Autodesk Inventor part; units mm, degrees
(part 3 of 11)
  arc A664 (23.2868, 30.3149) -> (23.2868, 30.2387) centre (23.2868, 30.2768) ccw
  arc A665 (26.162, 30.2387) -> (26.162, 30.3149) centre (26.162, 30.2768) ccw
  line L333 (27.1241, 30.7326) -> (21.4917, 28.6469)
  arc A666 (21.4537, 28.6494) -> (21.5298, 28.6444) centre (21.4917, 28.6469) ccw
  arc A667 (27.1241, 30.6945) -> (27.1241, 30.7707) centre (27.1241, 30.7326) ccw
  line L334 (26.162, 30.4292) -> (23.5117, 30.4292)
  arc A668 (23.5117, 30.4673) -> (23.5117, 30.3911) centre (23.5117, 30.4292) ccw
  arc A669 (26.162, 30.3911) -> (26.162, 30.4673) centre (26.162, 30.4292) ccw
  line L335 (26.8955, 30.6777) -> (26.7391, 28.3014)
  arc A670 (26.701, 28.3039) -> (26.7771, 28.2989) centre (26.7391, 28.3014) ccw
  arc A671 (26.8955, 30.6396) -> (26.8955, 30.7158) centre (26.8955, 30.6777) ccw
  line L336 (26.162, 30.5816) -> (23.7661, 30.5816)
  arc A672 (23.7661, 30.6197) -> (23.7661, 30.5435) centre (23.7661, 30.5816) ccw
  arc A673 (26.162, 30.5435) -> (26.162, 30.6197) centre (26.162, 30.5816) ccw
  line L337 (26.724, 30.3927) -> (26.587, 28.3115)
  arc A674 (26.549, 28.314) -> (26.625, 28.309) centre (26.587, 28.3115) ccw
  arc A675 (26.724, 30.3546) -> (26.724, 30.4308) centre (26.724, 30.3927) ccw
  line L338 (26.162, 30.734) -> (24.067, 30.734)
  arc A676 (24.067, 30.7721) -> (24.067, 30.6959) centre (24.067, 30.734) ccw
  arc A677 (26.162, 30.6959) -> (26.162, 30.7721) centre (26.162, 30.734) ccw
  line L339 (26.5493, 30.0586) -> (26.4349, 28.3215)
  arc A678 (26.3969, 28.324) -> (26.4729, 28.319) centre (26.4349, 28.3215) ccw
  arc A679 (26.5493, 30.0205) -> (26.5493, 30.0967) centre (26.5493, 30.0586) ccw
  line L340 (26.162, 30.8864) -> (24.4226, 30.8864)
  arc A680 (24.4226, 30.9245) -> (24.4226, 30.8483) centre (24.4226, 30.8864) ccw
  arc A681 (26.162, 30.8483) -> (26.162, 30.9245) centre (26.162, 30.8864) ccw
  line L341 (26.3694, 29.6455) -> (26.2829, 28.3315)
  arc A682 (26.2448, 28.334) -> (26.3209, 28.329) centre (26.2829, 28.3315) ccw
  arc A683 (26.3694, 29.6074) -> (26.3694, 29.6836) centre (26.3694, 29.6455) ccw
  line L342 (26.162, 31.0388) -> (24.8504, 31.0388)
  arc A684 (24.8504, 31.0769) -> (24.8504, 31.0007) centre (24.8504, 31.0388) ccw
  arc A685 (26.162, 31.0007) -> (26.162, 31.0769) centre (26.162, 31.0388) ccw
  line L343 (26.1708, 28.9489) -> (26.1308, 28.3415)
  arc A686 (26.0928, 28.344) -> (26.1688, 28.339) centre (26.1308, 28.3415) ccw
  arc A687 (26.1708, 28.9108) -> (26.1708, 28.987) centre (26.1708, 28.9489) ccw
  line L344 (26.162, 31.1912) -> (25.5924, 31.1912)
  arc A688 (25.5924, 31.2293) -> (25.5924, 31.1531) centre (25.5924, 31.1912) ccw
  arc A689 (26.162, 31.1531) -> (26.162, 31.2293) centre (26.162, 31.1912) ccw
  line L345 (26.0801, 28.3448) -> (26.177, 28.9906)
  arc A690 (26.2147, 28.9849) -> (26.1802, 29.0285) centre (26.177, 28.9906) ccw
  arc A691 (26.0833, 28.3828) -> (26.0769, 28.3069) centre (26.0801, 28.3448) ccw
  line L346 (26.177, 28.9906) -> (26.3574, 29.6181)
  arc A692 (26.394, 29.6076) -> (26.3655, 29.6553) centre (26.3574, 29.6181) ccw
  arc A693 (26.1404, 29.0011) -> (26.1689, 28.9533) centre (26.177, 28.9906) ccw
  line L347 (26.3574, 29.6181) -> (26.6182, 30.2168)
  arc A694 (26.6053, 30.1809) -> (26.6311, 30.2526) centre (26.6182, 30.2168) ccw
  arc A695 (26.3225, 29.6333) -> (26.3445, 29.5823) centre (26.3574, 29.6181) ccw
  line L348 (26.6182, 30.2168) -> (26.9548, 30.7763)
  arc A696 (26.9374, 30.7424) -> (26.9723, 30.8101) centre (26.9548, 30.7763) ccw
  arc A697 (26.6356, 30.2506) -> (26.6007, 30.1829) centre (26.6182, 30.2168) ccw
  line L349 (26.9548, 30.7763) -> (29.3598, 30.1565)
  arc A698 (29.3381, 30.1252) -> (29.3815, 30.1878) centre (29.3598, 30.1565) ccw
  arc A699 (26.9766, 30.8075) -> (26.9331, 30.745) centre (26.9548, 30.7763) ccw
  line L350 (29.3598, 30.1565) -> (29.843, 29.7173)
  arc A700 (29.8174, 29.6891) -> (29.8686, 29.7455) centre (29.843, 29.7173) ccw
  arc A701 (29.3854, 30.1847) -> (29.3342, 30.1283) centre (29.3598, 30.1565) ccw
  line L351 (29.843, 29.7173) -> (30.2647, 29.2188)
  arc A702 (30.2356, 29.1942) -> (30.2938, 29.2434) centre (30.2647, 29.2188) ccw
  arc A703 (29.8721, 29.7419) -> (29.8139, 29.6927) centre (29.843, 29.7173) ccw
  line L352 (30.2647, 29.2188) -> (30.6178, 28.6694)
  arc A704 (30.5857, 28.6489) -> (30.6498, 28.6901) centre (30.6178, 28.6694) ccw
  arc A705 (30.2968, 29.2394) -> (30.2327, 29.1982) centre (30.2647, 29.2188) ccw
  line L353 (30.6178, 28.6694) -> (30.8961, 28.0788)
  arc A706 (30.8616, 28.0625) -> (30.9306, 28.095) centre (30.8961, 28.0788) ccw
  arc A707 (30.6522, 28.6857) -> (30.5833, 28.6532) centre (30.6178, 28.6694) ccw
  line L354 (30.8961, 28.0788) -> (31.0949, 27.4568)
  arc A708 (31.0586, 27.4452) -> (31.1312, 27.4684) centre (31.0949, 27.4568) ccw
  arc A709 (30.9324, 28.0903) -> (30.8598, 28.0672) centre (30.8961, 28.0788) ccw
  line L355 (31.0949, 27.4568) -> (31.2111, 26.8142)
  arc A710 (31.1736, 26.8075) -> (31.2486, 26.821) centre (31.2111, 26.8142) ccw
  arc A711 (31.1324, 27.4636) -> (31.0574, 27.45) centre (31.0949, 27.4568) ccw
  line L356 (31.2111, 26.8142) -> (31.2392, 26.1619)
  arc A712 (31.2012, 26.1601) -> (31.2773, 26.1637) centre (31.2392, 26.1619) ccw
  arc A713 (31.2491, 26.8161) -> (31.173, 26.8124) centre (31.2111, 26.8142) ccw
  line L357 (31.2392, 26.1619) -> (31.2053, 25.5496)
  arc A714 (31.1673, 25.5519) -> (31.2433, 25.5473) centre (31.2053, 25.5496) ccw
  arc A715 (31.2773, 26.1596) -> (31.2012, 26.1642) centre (31.2392, 26.1619) ccw
  line L358 (31.2053, 25.5496) -> (31.0945, 24.9462)
  arc A716 (31.0569, 24.9531) -> (31.1319, 24.9394) centre (31.0944, 24.9463) ccw
  arc A717 (31.2428, 25.5427) -> (31.1678, 25.5565) centre (31.2053, 25.5496) ccw
  line L359 (31.0945, 24.9462) -> (30.9118, 24.3606)
  arc A718 (30.8754, 24.372) -> (30.9482, 24.3493) centre (30.9118, 24.3606) ccw
  arc A719 (31.1309, 24.9349) -> (31.0581, 24.9576) centre (31.0945, 24.9462) ccw
  line L360 (30.9118, 24.3606) -> (30.6601, 23.8012)
  arc A720 (30.6253, 23.8168) -> (30.6948, 23.7856) centre (30.6601, 23.8012) ccw
  arc A721 (30.9465, 24.345) -> (30.877, 24.3763) centre (30.9118, 24.3606) ccw
  line L361 (30.6601, 23.8012) -> (30.3428, 23.2762)
  arc A722 (30.3102, 23.2959) -> (30.3754, 23.2565) centre (30.3428, 23.2762) ccw
  arc A723 (30.6927, 23.7815) -> (30.6275, 23.8209) centre (30.6601, 23.8012) ccw
  line L362 (30.3428, 23.2762) -> (29.9645, 22.7933)
  arc A724 (29.9345, 22.8168) -> (29.9945, 22.7698) centre (29.9645, 22.7933) ccw
  arc A725 (30.3728, 23.2527) -> (30.3128, 23.2997) centre (30.3428, 23.2762) ccw
  line L363 (29.9645, 22.7933) -> (29.5307, 22.3596)
  arc A726 (29.5037, 22.3865) -> (29.5576, 22.3326) centre (29.5307, 22.3596) ccw
  arc A727 (29.9914, 22.7664) -> (29.9375, 22.8203) centre (29.9645, 22.7933) ccw
  line L364 (29.5307, 22.3596) -> (29.0478, 21.9812)
  arc A728 (29.0243, 22.0112) -> (29.0713, 21.9512) centre (29.0478, 21.9812) ccw
  arc A729 (29.5542, 22.3296) -> (29.5072, 22.3896) centre (29.5307, 22.3596) ccw
  line L365 (29.0478, 21.9812) -> (28.5228, 21.6639)
  arc A730 (28.5031, 21.6965) -> (28.5425, 21.6313) centre (28.5228, 21.6639) ccw
  arc A731 (29.0675, 21.9486) -> (29.0281, 22.0138) centre (29.0478, 21.9812) ccw
  line L366 (28.5228, 21.6639) -> (27.9634, 21.4121)
  arc A732 (27.9478, 21.4469) -> (27.9791, 21.3774) centre (27.9634, 21.4121) ccw
  arc A733 (28.5384, 21.6291) -> (28.5072, 21.6986) centre (28.5228, 21.6639) ccw
  line L367 (27.9634, 21.4121) -> (27.3777, 21.2296)
  arc A734 (27.3664, 21.266) -> (27.3891, 21.1933) centre (27.3777, 21.2296) ccw
  arc A735 (27.9747, 21.3758) -> (27.9521, 21.4485) centre (27.9634, 21.4121) ccw
  line L368 (27.3777, 21.2296) -> (26.7743, 21.119)
  arc A736 (26.7675, 21.1565) -> (26.7812, 21.0816) centre (26.7743, 21.119) ccw
  arc A737 (27.3846, 21.1921) -> (27.3709, 21.2671) centre (27.3777, 21.2296) ccw
  line L369 (26.7743, 21.119) -> (26.162, 21.082)
  arc A738 (26.1597, 21.12) -> (26.1643, 21.044) centre (26.162, 21.082) ccw
  arc A739 (26.7766, 21.081) -> (26.772, 21.1571) centre (26.7743, 21.119) ccw
  line L370 (26.162, 21.082) -> (25.5497, 21.119)
  arc A740 (25.552, 21.1571) -> (25.5474, 21.081) centre (25.5497, 21.119) ccw
  arc A741 (26.1597, 21.044) -> (26.1643, 21.12) centre (26.162, 21.082) ccw
  line L371 (25.5497, 21.119) -> (24.9463, 21.2296)
  arc A742 (24.9531, 21.2671) -> (24.9394, 21.1921) centre (24.9463, 21.2296) ccw
  arc A743 (25.5428, 21.0816) -> (25.5565, 21.1565) centre (25.5497, 21.119) ccw
  line L372 (24.9463, 21.2296) -> (24.3606, 21.4121)
  arc A744 (24.3719, 21.4485) -> (24.3493, 21.3758) centre (24.3606, 21.4121) ccw
  arc A745 (24.935, 21.1933) -> (24.9576, 21.266) centre (24.9463, 21.2296) ccw
  line L373 (24.3606, 21.4121) -> (23.8012, 21.6639)
  arc A746 (23.8168, 21.6986) -> (23.7856, 21.6291) centre (23.8012, 21.6639) ccw
  arc A747 (24.345, 21.3774) -> (24.3763, 21.4469) centre (24.3606, 21.4121) ccw
  line L374 (23.8012, 21.6639) -> (23.2762, 21.9812)
  arc A748 (23.2959, 22.0138) -> (23.2565, 21.9486) centre (23.2762, 21.9812) ccw
  arc A749 (23.7815, 21.6313) -> (23.8209, 21.6965) centre (23.8012, 21.6639) ccw
  line L375 (23.2762, 21.9812) -> (22.7933, 22.3596)
  arc A750 (22.8168, 22.3896) -> (22.7698, 22.3296) centre (22.7933, 22.3596) ccw
  arc A751 (23.2527, 21.9512) -> (23.2997, 22.0112) centre (23.2762, 21.9812) ccw
  line L376 (22.7933, 22.3596) -> (22.3596, 22.7933)
  arc A752 (22.3865, 22.8203) -> (22.3326, 22.7664) centre (22.3596, 22.7933) ccw
  arc A753 (22.7664, 22.3326) -> (22.8203, 22.3865) centre (22.7933, 22.3596) ccw
  line L377 (22.3596, 22.7933) -> (21.9812, 23.2762)
  arc A754 (22.0112, 23.2997) -> (21.9512, 23.2527) centre (21.9812, 23.2762) ccw
  arc A755 (22.3296, 22.7698) -> (22.3896, 22.8168) centre (22.3596, 22.7933) ccw
  line L378 (21.9812, 23.2762) -> (21.6639, 23.8012)
  arc A756 (21.6965, 23.8209) -> (21.6313, 23.7815) centre (21.6639, 23.8012) ccw
  arc A757 (21.9486, 23.2565) -> (22.0139, 23.2959) centre (21.9812, 23.2762) ccw
  line L379 (21.6639, 23.8012) -> (21.4121, 24.3606)
  arc A758 (21.4469, 24.3763) -> (21.3774, 24.345) centre (21.4121, 24.3606) ccw
  arc A759 (21.6291, 23.7856) -> (21.6986, 23.8168) centre (21.6639, 23.8012) ccw
  line L380 (21.4121, 24.3606) -> (21.2296, 24.9463)
  arc A760 (21.266, 24.9576) -> (21.1933, 24.935) centre (21.2296, 24.9463) ccw
  arc A761 (21.3758, 24.3493) -> (21.4485, 24.3719) centre (21.4121, 24.3606) ccw
  line L381 (21.2296, 24.9463) -> (21.119, 25.5497)
  arc A762 (21.1565, 25.5565) -> (21.0816, 25.5428) centre (21.119, 25.5497) ccw
  arc A763 (21.1921, 24.9394) -> (21.2671, 24.9531) centre (21.2296, 24.9463) ccw
  line L382 (21.119, 25.5497) -> (21.082, 26.162)
  arc A764 (21.12, 26.1643) -> (21.044, 26.1597) centre (21.082, 26.162) ccw
  arc A765 (21.081, 25.5474) -> (21.1571, 25.552) centre (21.119, 25.5497) ccw
  line L383 (21.082, 26.162) -> (21.1406, 26.8194)
  arc A766 (21.1786, 26.816) -> (21.1027, 26.8228) centre (21.1406, 26.8194) ccw
  arc A767 (21.0441, 26.1654) -> (21.1199, 26.1586) centre (21.082, 26.162) ccw
  line L384 (21.1406, 26.8194) -> (21.2818, 27.464)
  arc A768 (21.319, 27.4559) -> (21.2446, 27.4722) centre (21.2818, 27.464) ccw
  arc A769 (21.1034, 26.8275) -> (21.1778, 26.8112) centre (21.1406, 26.8194) ccw
  line L385 (21.2818, 27.464) -> (21.5033, 28.0857)
  arc A770 (21.5392, 28.073) -> (21.4674, 28.0985) centre (21.5033, 28.0857) ccw
  arc A771 (21.2459, 27.4768) -> (21.3177, 27.4513) centre (21.2818, 27.464) ccw
  line L386 (21.5033, 28.0857) -> (21.8015, 28.6745)
  arc A772 (21.8355, 28.6573) -> (21.7675, 28.6917) centre (21.8015, 28.6745) ccw
  arc A773 (21.4693, 28.103) -> (21.5373, 28.0685) centre (21.5033, 28.0857) ccw
  line L387 (21.8015, 28.6745) -> (22.1716, 29.2209)
  arc A774 (22.2032, 29.1995) -> (22.1401, 29.2422) centre (22.1716, 29.2209) ccw
  arc A775 (21.7699, 28.6959) -> (21.833, 28.6532) centre (21.8015, 28.6745) ccw
  line L388 (22.1716, 29.2209) -> (22.6078, 29.7162)
  arc A776 (22.6364, 29.691) -> (22.5793, 29.7413) centre (22.6078, 29.7162) ccw
  arc A777 (22.143, 29.2461) -> (22.2002, 29.1957) centre (22.1716, 29.2209) ccw
  line L389 (22.6078, 29.7162) -> (23.1031, 30.1524)
  arc A778 (23.1283, 30.1238) -> (23.0779, 30.181) centre (23.1031, 30.1524) ccw
  arc A779 (22.5827, 29.7447) -> (22.633, 29.6876) centre (22.6078, 29.7162) ccw
  line L390 (23.1031, 30.1524) -> (23.6495, 30.5225)
  arc A780 (23.6708, 30.491) -> (23.6281, 30.5541) centre (23.6495, 30.5225) ccw
  arc A781 (23.0817, 30.1839) -> (23.1245, 30.1208) centre (23.1031, 30.1524) ccw
  line L391 (23.6495, 30.5225) -> (24.2383, 30.8207)
  arc A782 (24.2555, 30.7867) -> (24.221, 30.8547) centre (24.2382, 30.8207) ccw
  arc A783 (23.6323, 30.5565) -> (23.6667, 30.4885) centre (23.6495, 30.5225) ccw
  line L392 (24.2383, 30.8207) -> (24.8599, 31.0422)
  arc A784 (24.8727, 31.0063) -> (24.8472, 31.0781) centre (24.8599, 31.0422) ccw
  arc A785 (24.2255, 30.8566) -> (24.251, 30.7848) centre (24.2382, 30.8207) ccw
  line L393 (24.8599, 31.0422) -> (25.5046, 31.1834)
  arc A786 (25.5128, 31.1462) -> (25.4965, 31.2206) centre (25.5046, 31.1834) ccw
  arc A787 (24.8518, 31.0794) -> (24.8681, 31.005) centre (24.8599, 31.0422) ccw
  line L394 (25.5046, 31.1834) -> (26.162, 31.242)
  arc A788 (26.1654, 31.2041) -> (26.1586, 31.28) centre (26.162, 31.242) ccw
  arc A789 (25.5012, 31.2213) -> (25.508, 31.1454) centre (25.5046, 31.1834) ccw
  line L395 (26.162, 31.242) -> (26.162, 29.972)
  arc A790 (26.1239, 29.972) -> (26.2001, 29.972) centre (26.162, 29.972) ccw
  arc A791 (26.2001, 31.242) -> (26.1239, 31.242) centre (26.162, 31.242) ccw
  line L396 (26.162, 29.972) -> (25.6365, 29.9526)
  arc A792 (25.6352, 29.9907) -> (25.638, 29.9145) centre (25.6366, 29.9526) ccw
  arc A793 (26.1634, 29.9339) -> (26.1606, 30.0101) centre (26.162, 29.972) ccw
  line L397 (25.6365, 29.9526) -> (25.1192, 29.8586)
  arc A794 (25.1124, 29.8961) -> (25.126, 29.8211) centre (25.1192, 29.8586) ccw
  arc A795 (25.6434, 29.9151) -> (25.6297, 29.9901) centre (25.6366, 29.9526) ccw
  line L398 (25.1192, 29.8586) -> (24.6206, 29.6919)
  arc A796 (24.6085, 29.7281) -> (24.6326, 29.6558) centre (24.6206, 29.6919) ccw
  arc A797 (25.1313, 29.8225) -> (25.1072, 29.8947) centre (25.1192, 29.8586) ccw
  line L399 (24.6206, 29.6919) -> (24.1507, 29.456)
  arc A798 (24.1336, 29.49) -> (24.1677, 29.4219) centre (24.1506, 29.456) ccw
  arc A799 (24.6376, 29.6579) -> (24.6035, 29.726) centre (24.6206, 29.6919) ccw
  line L400 (24.1507, 29.456) -> (23.7191, 29.1556)
  arc A800 (23.6974, 29.1868) -> (23.7409, 29.1243) centre (23.7191, 29.1556) ccw
  arc A801 (24.1724, 29.4247) -> (24.1289, 29.4873) centre (24.1507, 29.456) ccw
  line L401 (23.7191, 29.1556) -> (23.3348, 28.7968)
  arc A802 (23.3087, 28.8247) -> (23.3607, 28.769) centre (23.3347, 28.7968) ccw
  arc A803 (23.7451, 29.1277) -> (23.6931, 29.1834) centre (23.7191, 29.1556) ccw
  line L402 (23.3348, 28.7968) -> (23.0053, 28.387)
  arc A804 (22.9756, 28.4109) -> (23.035, 28.3631) centre (23.0053, 28.387) ccw
  arc A805 (23.3644, 28.773) -> (23.305, 28.8207) centre (23.3347, 28.7968) ccw
  line L403 (23.0053, 28.387) -> (22.7376, 27.9345)
  arc A806 (22.7048, 27.9539) -> (22.7704, 27.9151) centre (22.7376, 27.9345) ccw
  arc A807 (23.0381, 28.3676) -> (22.9725, 28.4064) centre (23.0053, 28.387) ccw
  line L404 (22.7376, 27.9345) -> (22.5369, 27.4485)
  arc A808 (22.5018, 27.463) -> (22.5722, 27.4339) centre (22.537, 27.4485) ccw
  arc A809 (22.7728, 27.92) -> (22.7024, 27.949) centre (22.7376, 27.9345) ccw
  line L405 (22.5369, 27.4485) -> (22.4076, 26.9389)
  arc A810 (22.3706, 26.9482) -> (22.4445, 26.9295) centre (22.4076, 26.9388) ccw
  arc A811 (22.5739, 27.4391) -> (22.5, 27.4579) centre (22.5369, 27.4485) ccw
  line L406 (22.4076, 26.9389) -> (22.352, 26.416)
  arc A812 (22.3141, 26.42) -> (22.3899, 26.412) centre (22.352, 26.416) ccw
  arc A813 (22.4454, 26.9348) -> (22.3697, 26.9429) centre (22.4076, 26.9388) ccw
  line L407 (22.352, 26.416) -> (22.352, 26.162)
  arc A814 (22.3139, 26.162) -> (22.3901, 26.162) centre (22.352, 26.162) ccw
  arc A815 (22.3901, 26.416) -> (22.3139, 26.416) centre (22.352, 26.416) ccw
  line L408 (22.352, 26.162) -> (22.3908, 25.6198)
  arc A816 (22.3528, 25.6171) -> (22.4288, 25.6225) centre (22.3908, 25.6198) ccw
  arc A817 (22.39, 26.1647) -> (22.314, 26.1593) centre (22.352, 26.162) ccw
  line L409 (22.3908, 25.6198) -> (22.5063, 25.0886)
  arc A818 (22.4691, 25.0805) -> (22.5436, 25.0967) centre (22.5063, 25.0886) ccw
  arc A819 (22.428, 25.6279) -> (22.3536, 25.6117) centre (22.3908, 25.6198) ccw
  line L410 (22.5063, 25.0886) -> (22.6963, 24.5793)
  arc A820 (22.6606, 24.566) -> (22.732, 24.5926) centre (22.6963, 24.5793) ccw
  arc A821 (22.542, 25.1019) -> (22.4706, 25.0753) centre (22.5063, 25.0886) ccw
  line L411 (22.6963, 24.5793) -> (22.9568, 24.1022)
  arc A822 (22.9234, 24.0839) -> (22.9903, 24.1204) centre (22.9568, 24.1022) ccw
  arc A823 (22.7297, 24.5975) -> (22.6629, 24.561) centre (22.6963, 24.5793) ccw
  line L412 (22.9568, 24.1022) -> (23.2827, 23.6671)
  arc A824 (23.2521, 23.6441) -> (23.3131, 23.6898) centre (23.2826, 23.667) ccw
  arc A825 (22.9873, 24.125) -> (22.9263, 24.0793) centre (22.9568, 24.1022) ccw
  line L413 (23.2827, 23.6671) -> (23.667, 23.2826)
  arc A826 (23.64, 23.2557) -> (23.6939, 23.3095) centre (23.667, 23.2826) ccw
  arc A827 (23.3095, 23.6939) -> (23.2557, 23.64) centre (23.2826, 23.667) ccw
  line L414 (23.667, 23.2826) -> (24.1022, 22.9568)
  arc A828 (24.0793, 22.9263) -> (24.125, 22.9873) centre (24.1022, 22.9568) ccw
  arc A829 (23.6898, 23.3131) -> (23.6441, 23.2521) centre (23.667, 23.2826) ccw
  line L415 (24.1022, 22.9568) -> (24.5793, 22.6963)
  arc A830 (24.561, 22.6629) -> (24.5975, 22.7297) centre (24.5793, 22.6963) ccw
  arc A831 (24.1204, 22.9903) -> (24.0839, 22.9234) centre (24.1022, 22.9568) ccw
  line L416 (24.5793, 22.6963) -> (25.0886, 22.5063)
  arc A832 (25.0753, 22.4706) -> (25.1019, 22.542) centre (25.0886, 22.5063) ccw
  arc A833 (24.5926, 22.732) -> (24.566, 22.6606) centre (24.5793, 22.6963) ccw
  line L417 (25.0886, 22.5063) -> (25.6198, 22.3908)
  arc A834 (25.6117, 22.3536) -> (25.6279, 22.428) centre (25.6198, 22.3908) ccw
  arc A835 (25.0967, 22.5436) -> (25.0805, 22.4691) centre (25.0886, 22.5063) ccw
  line L418 (25.6198, 22.3908) -> (26.162, 22.352)
  arc A836 (26.1593, 22.314) -> (26.1647, 22.39) centre (26.162, 22.352) ccw
  arc A837 (25.6225, 22.4288) -> (25.6171, 22.3528) centre (25.6198, 22.3908) ccw
  line L419 (26.162, 22.352) -> (26.7042, 22.3908)
  arc A838 (26.7069, 22.3528) -> (26.7015, 22.4288) centre (26.7042, 22.3908) ccw
  arc A839 (26.1593, 22.39) -> (26.1647, 22.314) centre (26.162, 22.352) ccw
  line L420 (26.7042, 22.3908) -> (27.2354, 22.5063)
  arc A840 (27.2435, 22.4691) -> (27.2273, 22.5436) centre (27.2354, 22.5063) ccw
  arc A841 (26.6961, 22.428) -> (26.7123, 22.3535) centre (26.7042, 22.3908) ccw
  line L421 (27.2354, 22.5063) -> (27.7447, 22.6963)
  arc A842 (27.758, 22.6606) -> (27.7314, 22.732) centre (27.7447, 22.6963) ccw
  arc A843 (27.2221, 22.542) -> (27.2487, 22.4706) centre (27.2354, 22.5063) ccw
  line L422 (27.7447, 22.6963) -> (28.2218, 22.9568)
  arc A844 (28.2401, 22.9234) -> (28.2036, 22.9903) centre (28.2218, 22.9568) ccw
  arc A845 (27.7265, 22.7297) -> (27.763, 22.6629) centre (27.7447, 22.6963) ccw
  line L423 (28.2218, 22.9568) -> (28.657, 23.2826)
  arc A846 (28.6799, 23.2521) -> (28.6342, 23.3131) centre (28.657, 23.2826) ccw
  arc A847 (28.199, 22.9873) -> (28.2447, 22.9263) centre (28.2218, 22.9568) ccw
  line L424 (28.657, 23.2826) -> (29.0414, 23.667)
  arc A848 (29.0683, 23.64) -> (29.0145, 23.6939) centre (29.0414, 23.667) ccw
  arc A849 (28.6301, 23.3095) -> (28.684, 23.2557) centre (28.657, 23.2826) ccw
  line L425 (29.0414, 23.667) -> (29.3672, 24.1022)
  arc A850 (29.3977, 24.0793) -> (29.3367, 24.125) centre (29.3672, 24.1022) ccw
  arc A851 (29.0109, 23.6898) -> (29.0719, 23.6441) centre (29.0414, 23.667) ccw
  line L426 (29.3672, 24.1022) -> (29.6277, 24.5793)
  arc A852 (29.6611, 24.561) -> (29.5943, 24.5975) centre (29.6277, 24.5793) ccw
  arc A853 (29.3337, 24.1204) -> (29.4006, 24.0839) centre (29.3672, 24.1022) ccw
  line L427 (29.6277, 24.5793) -> (29.8177, 25.0886)
  arc A854 (29.8534, 25.0753) -> (29.782, 25.1019) centre (29.8177, 25.0886) ccw
  arc A855 (29.592, 24.5926) -> (29.6634, 24.566) centre (29.6277, 24.5793) ccw
  line L428 (29.8177, 25.0886) -> (29.9332, 25.6198)
  arc A856 (29.9704, 25.6117) -> (29.896, 25.6279) centre (29.9332, 25.6198) ccw
  arc A857 (29.7804, 25.0967) -> (29.8549, 25.0805) centre (29.8177, 25.0886) ccw
  line L429 (29.9332, 25.6198) -> (29.972, 26.162)
  arc A858 (30.01, 26.1593) -> (29.934, 26.1647) centre (29.972, 26.162) ccw
  arc A859 (29.8952, 25.6225) -> (29.9712, 25.6171) centre (29.9332, 25.6198) ccw
  line L430 (29.972, 26.162) -> (29.9518, 26.6485)
  arc A860 (29.9898, 26.65) -> (29.9137, 26.6469) centre (29.9518, 26.6485) ccw
  arc A861 (29.9339, 26.1604) -> (30.0101, 26.1636) centre (29.972, 26.162) ccw
  line L431 (29.9518, 26.6485) -> (29.8682, 27.1281)
  arc A862 (29.9058, 27.1347) -> (29.8307, 27.1216) centre (29.8682, 27.1281) ccw
  arc A863 (29.9142, 26.6419) -> (29.9893, 26.655) centre (29.9518, 26.6485) ccw
  line L432 (29.8682, 27.1281) -> (29.7228, 27.5928)
  arc A864 (29.7591, 27.6042) -> (29.6864, 27.5814) centre (29.7228, 27.5928) ccw
  arc A865 (29.8318, 27.1167) -> (29.9046, 27.1395) centre (29.8682, 27.1281) ccw
  line L433 (29.7228, 27.5928) -> (29.5179, 28.0345)
  arc A866 (29.5525, 28.0505) -> (29.4834, 28.0184) centre (29.5179, 28.0345) ccw
  arc A867 (29.6882, 27.5767) -> (29.7574, 27.6088) centre (29.7228, 27.5928) ccw
  line L434 (29.5179, 28.0345) -> (29.2572, 28.4456)
  arc A868 (29.2893, 28.466) -> (29.225, 28.4252) centre (29.2572, 28.4456) ccw
  arc A869 (29.4857, 28.0141) -> (29.5501, 28.0549) centre (29.5179, 28.0345) ccw
  line L435 (29.2572, 28.4456) -> (28.945, 28.8193)
  arc A870 (28.9742, 28.8437) -> (28.9157, 28.7948) centre (28.945, 28.8193) ccw
  arc A871 (29.2279, 28.4212) -> (29.2864, 28.4701) centre (29.2572, 28.4456) ccw
  line L436 (28.945, 28.8193) -> (28.5867, 29.1489)
  arc A872 (28.6125, 29.177) -> (28.5609, 29.1209) centre (28.5867, 29.1489) ccw
  arc A873 (28.9192, 28.7912) -> (28.9708, 28.8473) centre (28.945, 28.8193) ccw
  line L437 (28.5867, 29.1489) -> (28.1884, 29.429)
  arc A874 (28.2104, 29.4602) -> (28.1665, 29.3979) centre (28.1884, 29.429) ccw
  arc A875 (28.5648, 29.1178) -> (28.6086, 29.1801) centre (28.5867, 29.1489) ccw
  line L438 (28.1884, 29.429) -> (27.757, 29.6547)
  arc A876 (27.7747, 29.6885) -> (27.7394, 29.621) centre (27.757, 29.6547) ccw
  arc A877 (28.1708, 29.3953) -> (28.2061, 29.4628) centre (28.1884, 29.429) ccw
  line L439 (27.757, 29.6547) -> (27.5599, 29.2096)
  arc A878 (27.313, 29.858) -> (27.2868, 29.7864) centre (27.2999, 29.8222) ccw
  arc A879 (27.7439, 29.619) -> (27.7702, 29.6905) centre (27.757, 29.6547) ccw
  line L440 (27.5599, 29.2096) -> (27.4225, 28.7424)
  arc A880 (27.4309, 28.7796) -> (27.4142, 28.7052) centre (27.4225, 28.7424) ccw
  arc A881 (27.5516, 29.1724) -> (27.5682, 29.2467) centre (27.5599, 29.2095) ccw
  line L441 (27.4225, 28.7424) -> (27.3473, 28.2614)
  arc A882 (27.3507, 28.2993) -> (27.3439, 28.2235) centre (27.3473, 28.2614) ccw
  arc A883 (27.4191, 28.7045) -> (27.4259, 28.7804) centre (27.4225, 28.7424) ccw
  line L442 (27.3473, 28.2614) -> (26.0801, 28.3448)
  arc A884 (26.1182, 28.3448) -> (26.042, 28.3448) centre (26.0801, 28.3448) ccw
  arc A885 (27.3092, 28.2614) -> (27.3775, 28.2847) centre (27.3473, 28.2614) ccw
  line L443 (26.8494, 21.1328) -> (25.4746, 21.1328)
  arc A886 (25.4746, 21.1709) -> (25.4746, 21.0947) centre (25.4746, 21.1328) ccw
  arc A887 (26.8494, 21.0947) -> (26.8494, 21.1709) centre (26.8494, 21.1328) ccw
  line L444 (27.5561, 21.2852) -> (24.7679, 21.2852)
  arc A888 (24.7679, 21.3233) -> (24.7679, 21.2471) centre (24.7679, 21.2852) ccw
  arc A889 (27.5561, 21.2471) -> (27.5561, 21.3233) centre (27.5561, 21.2852) ccw
  line L445 (28.02, 21.4376) -> (24.304, 21.4376)
  arc A890 (24.304, 21.4757) -> (24.304, 21.3995) centre (24.304, 21.4376) ccw
  arc A891 (28.02, 21.3995) -> (28.02, 21.4757) centre (28.02, 21.4376) ccw
  line L446 (28.3587, 21.59) -> (23.9654, 21.59)
  arc A892 (23.9654, 21.6281) -> (23.9654, 21.5519) centre (23.9654, 21.59) ccw
  arc A893 (28.3587, 21.5519) -> (28.3587, 21.6281) centre (28.3587, 21.59) ccw
  line L447 (28.6527, 21.7424) -> (23.6713, 21.7424)
  arc A894 (23.6713, 21.7805) -> (23.6713, 21.7043) centre (23.6713, 21.7424) ccw
  arc A895 (28.6527, 21.7043) -> (28.6527, 21.7805) centre (28.6527, 21.7424) ccw
  line L448 (28.9048, 21.8948) -> (23.4192, 21.8948)
  arc A896 (23.4192, 21.9329) -> (23.4192, 21.8567) centre (23.4192, 21.8948) ccw
  arc A897 (28.9048, 21.8567) -> (28.9048, 21.9329) centre (28.9048, 21.8948) ccw
  line L449 (29.132, 22.0472) -> (23.1921, 22.0471)
  arc A898 (23.1921, 22.0852) -> (23.1921, 22.009) centre (23.1921, 22.0471) ccw
  arc A899 (29.132, 22.0091) -> (29.132, 22.0853) centre (29.132, 22.0472) ccw
  line L450 (29.3265, 22.1996) -> (22.9975, 22.1996)
  arc A900 (22.9975, 22.2377) -> (22.9975, 22.1615) centre (22.9975, 22.1996) ccw
  arc A901 (29.3265, 22.1615) -> (29.3265, 22.2377) centre (29.3265, 22.1996) ccw
  line L451 (29.521, 22.352) -> (26.162, 22.352)
  arc A902 (26.162, 22.3901) -> (26.162, 22.3139) centre (26.162, 22.352) ccw
  arc A903 (29.521, 22.3139) -> (29.521, 22.3901) centre (29.521, 22.352) ccw
  line L452 (26.162, 22.352) -> (22.803, 22.352)
  arc A904 (22.803, 22.3901) -> (22.803, 22.3139) centre (22.803, 22.352) ccw
  arc A905 (26.162, 22.3139) -> (26.162, 22.3901) centre (26.162, 22.352) ccw
  line L453 (29.6755, 22.5044) -> (27.2265, 22.5044)
  arc A906 (27.2265, 22.5425) -> (27.2265, 22.4663) centre (27.2265, 22.5044) ccw
  arc A907 (29.6755, 22.4663) -> (29.6755, 22.5425) centre (29.6755, 22.5044) ccw
  line L454 (25.0975, 22.5044) -> (22.6485, 22.5044)
  arc A908 (22.6485, 22.5425) -> (22.6485, 22.4663) centre (22.6485, 22.5044) ccw
  arc A909 (25.0975, 22.4663) -> (25.0975, 22.5425) centre (25.0975, 22.5044) ccw
  line L455 (29.8279, 22.6568) -> (27.6388, 22.6568)
  arc A910 (27.6388, 22.6949) -> (27.6388, 22.6187) centre (27.6388, 22.6568) ccw
  arc A911 (29.8279, 22.6187) -> (29.8279, 22.6949) centre (29.8279, 22.6568) ccw
  line L456 (24.6852, 22.6568) -> (22.4961, 22.6568)
  arc A912 (22.4961, 22.6949) -> (22.4961, 22.6187) centre (22.4961, 22.6568) ccw
  arc A913 (24.6852, 22.6187) -> (24.6852, 22.6949) centre (24.6852, 22.6568) ccw
  line L457 (29.9769, 22.8092) -> (27.9515, 22.8092)
  arc A914 (27.9515, 22.8473) -> (27.9515, 22.7711) centre (27.9515, 22.8092) ccw
  arc A915 (29.9769, 22.7711) -> (29.9769, 22.8473) centre (29.9769, 22.8092) ccw
  line L458 (24.3725, 22.8092) -> (22.3471, 22.8092)
  arc A916 (22.3471, 22.8473) -> (22.3471, 22.7711) centre (22.3471, 22.8092) ccw
  arc A917 (24.3725, 22.7711) -> (24.3725, 22.8473) centre (24.3725, 22.8092) ccw
  line L459 (30.0963, 22.9616) -> (28.2282, 22.9616)
  arc A918 (28.2282, 22.9997) -> (28.2282, 22.9235) centre (28.2282, 22.9616) ccw
  arc A919 (30.0963, 22.9235) -> (30.0963, 22.9997) centre (30.0963, 22.9616) ccw
  line L460 (24.0958, 22.9616) -> (22.2277, 22.9616)
  arc A920 (22.2277, 22.9997) -> (22.2277, 22.9235) centre (22.2277, 22.9616) ccw
  arc A921 (24.0958, 22.9235) -> (24.0958, 22.9997) centre (24.0958, 22.9616) ccw
  line L461 (30.2157, 23.114) -> (28.4318, 23.114)
  arc A922 (28.4318, 23.1521) -> (28.4318, 23.0759) centre (28.4318, 23.114) ccw
  arc A923 (30.2157, 23.0759) -> (30.2157, 23.1521) centre (30.2157, 23.114) ccw
  line L462 (23.8922, 23.114) -> (22.1083, 23.114)
  arc A924 (22.1083, 23.1521) -> (22.1083, 23.0759) centre (22.1083, 23.114) ccw
  arc A925 (23.8922, 23.0759) -> (23.8922, 23.1521) centre (23.8922, 23.114) ccw
  line L463 (30.3351, 23.2664) -> (28.6354, 23.2664)
  arc A926 (28.6354, 23.3045) -> (28.6354, 23.2283) centre (28.6354, 23.2664) ccw
  arc A927 (30.3351, 23.2283) -> (30.3351, 23.3045) centre (30.3351, 23.2664) ccw
  line L464 (23.6886, 23.2664) -> (21.9889, 23.2664)
  arc A928 (21.9889, 23.3045) -> (21.9889, 23.2283) centre (21.9889, 23.2664) ccw
  arc A929 (23.6886, 23.2283) -> (23.6886, 23.3045) centre (23.6886, 23.2664) ccw
  line L465 (30.429, 23.4188) -> (28.7933, 23.4186)
  arc A930 (28.7933, 23.4567) -> (28.7933, 23.3805) centre (28.7933, 23.4186) ccw
  arc A931 (30.429, 23.3807) -> (30.429, 23.4569) centre (30.429, 23.4188) ccw
  line L466 (23.5308, 23.4188) -> (21.8951, 23.4188)
  arc A932 (21.8951, 23.4569) -> (21.8951, 23.3807) centre (21.8951, 23.4188) ccw
  arc A933 (23.5308, 23.3807) -> (23.5308, 23.4569) centre (23.5308, 23.4188) ccw
  line L467 (30.5211, 23.5712) -> (28.9456, 23.571)
  arc A934 (28.9456, 23.6091) -> (28.9456, 23.5329) centre (28.9456, 23.571) ccw
  arc A935 (30.5211, 23.5331) -> (30.5211, 23.6093) centre (30.5211, 23.5712) ccw
  line L468 (23.3784, 23.5712) -> (21.8029, 23.5712)
  arc A936 (21.8029, 23.6093) -> (21.8029, 23.5331) centre (21.8029, 23.5712) ccw
  arc A937 (23.3784, 23.5331) -> (23.3784, 23.6093) centre (23.3784, 23.5712) ccw
  line L469 (30.6132, 23.7236) -> (29.0838, 23.7236)
  arc A938 (29.0838, 23.7617) -> (29.0838, 23.6855) centre (29.0838, 23.7236) ccw
  arc A939 (30.6132, 23.6855) -> (30.6132, 23.7617) centre (30.6132, 23.7236) ccw
  line L470 (23.2403, 23.7237) -> (21.7108, 23.7236)
  arc A940 (21.7108, 23.7617) -> (21.7108, 23.6855) centre (21.7108, 23.7236) ccw
  arc A941 (23.2403, 23.6856) -> (23.2403, 23.7618) centre (23.2403, 23.7237) ccw
  line L471 (30.6937, 23.876) -> (29.1979, 23.8758)
  arc A942 (29.1979, 23.9139) -> (29.1979, 23.8377) centre (29.1979, 23.8758) ccw
  arc A943 (30.6937, 23.8379) -> (30.6937, 23.9141) centre (30.6937, 23.876) ccw
  line L472 (23.1261, 23.876) -> (21.6302, 23.876)
  arc A944 (21.6302, 23.9141) -> (21.6302, 23.8379) centre (21.6302, 23.876) ccw
  arc A945 (23.1261, 23.8379) -> (23.1261, 23.9141) centre (23.1261, 23.876) ccw
  line L473 (30.7623, 24.0284) -> (29.312, 24.0284)
  arc A946 (29.312, 24.0665) -> (29.312, 23.9903) centre (29.312, 24.0284) ccw
  arc A947 (30.7623, 23.9903) -> (30.7623, 24.0665) centre (30.7623, 24.0284) ccw
  arc A948 (21.5616, 24.0665) -> (21.5616, 23.9903) centre (21.5616, 24.0284) ccw
  arc A949 (23.0121, 23.9903) -> (23.0121, 24.0665) centre (23.0121, 24.0284) ccw
  line L474 (30.8309, 24.1808) -> (29.4101, 24.1808)
  arc A950 (29.4101, 24.2189) -> (29.4101, 24.1427) centre (29.4101, 24.1808) ccw
  arc A951 (30.8309, 24.1427) -> (30.8309, 24.2189) centre (30.8309, 24.1808) ccw
  line L475 (22.9139, 24.1808) -> (21.4931, 24.1808)
  arc A952 (21.4931, 24.2189) -> (21.4931, 24.1427) centre (21.4931, 24.1808) ccw
  arc A953 (22.9139, 24.1427) -> (22.9139, 24.2189) centre (22.9139, 24.1808) ccw
  line L476 (30.8996, 24.3332) -> (29.4933, 24.3332)
  arc A954 (29.4933, 24.3713) -> (29.4933, 24.2951) centre (29.4933, 24.3332) ccw
  arc A955 (30.8996, 24.2951) -> (30.8996, 24.3713) centre (30.8996, 24.3332) ccw
  line L477 (22.8307, 24.3332) -> (21.4245, 24.3332)
  arc A956 (21.4245, 24.3713) -> (21.4245, 24.2951) centre (21.4245, 24.3332) ccw
  arc A957 (22.8307, 24.2951) -> (22.8307, 24.3713) centre (22.8307, 24.3332) ccw
  line L478 (30.9508, 24.4856) -> (29.5765, 24.4856)
  arc A958 (29.5765, 24.5237) -> (29.5765, 24.4475) centre (29.5765, 24.4856) ccw
  arc A959 (30.9508, 24.4475) -> (30.9508, 24.5237) centre (30.9508, 24.4856) ccw
  line L479 (22.7474, 24.4856) -> (21.3732, 24.4857)
  arc A960 (21.3732, 24.5238) -> (21.3732, 24.4476) centre (21.3732, 24.4857) ccw
  arc A961 (22.7474, 24.4475) -> (22.7474, 24.5237) centre (22.7474, 24.4856) ccw
  line L480 (30.9983, 24.638) -> (29.6496, 24.638)
  arc A962 (29.6496, 24.6761) -> (29.6496, 24.5999) centre (29.6496, 24.638) ccw
  arc A963 (30.9983, 24.5999) -> (30.9983, 24.6761) centre (30.9983, 24.638) ccw
  line L481 (22.6744, 24.638) -> (21.3257, 24.638)
  arc A964 (21.3257, 24.6761) -> (21.3257, 24.5999) centre (21.3257, 24.638) ccw
  arc A965 (22.6744, 24.5999) -> (22.6744, 24.6761) centre (22.6744, 24.638) ccw
  line L482 (31.0459, 24.7904) -> (29.7064, 24.7904)
  arc A966 (29.7064, 24.8285) -> (29.7064, 24.7523) centre (29.7064, 24.7904) ccw
  arc A967 (31.0459, 24.7523) -> (31.0459, 24.8285) centre (31.0459, 24.7904) ccw
  line L483 (22.6176, 24.7904) -> (21.2782, 24.7904)
  arc A968 (21.2782, 24.8285) -> (21.2782, 24.7523) centre (21.2782, 24.7904) ccw
  arc A969 (22.6176, 24.7523) -> (22.6176, 24.8285) centre (22.6176, 24.7904) ccw
  line L484 (31.0933, 24.9428) -> (29.7633, 24.9428)
  arc A970 (29.7633, 24.9809) -> (29.7633, 24.9047) centre (29.7633, 24.9428) ccw
  arc A971 (31.0933, 24.9047) -> (31.0933, 24.9809) centre (31.0933, 24.9428) ccw
  line L485 (22.5607, 24.9428) -> (21.2307, 24.9428)
  arc A972 (21.2307, 24.9809) -> (21.2307, 24.9047) centre (21.2307, 24.9428) ccw
  arc A973 (22.5607, 24.9047) -> (22.5607, 24.9809) centre (22.5607, 24.9428) ccw
  line L486 (31.1217, 25.0952) -> (29.8191, 25.0952)
  arc A974 (29.8191, 25.1333) -> (29.8191, 25.0571) centre (29.8191, 25.0952) ccw
  arc A975 (31.1217, 25.0571) -> (31.1217, 25.1333) centre (31.1217, 25.0952) ccw
  line L487 (22.5049, 25.0952) -> (21.2023, 25.0952)
  arc A976 (21.2023, 25.1333) -> (21.2023, 25.0571) centre (21.2023, 25.0952) ccw
  arc A977 (22.5049, 25.0571) -> (22.5049, 25.1333) centre (22.5049, 25.0952) ccw
  line L488 (31.1498, 25.2475) -> (29.8523, 25.2476)
  arc A978 (29.8523, 25.2857) -> (29.8523, 25.2095) centre (29.8523, 25.2476) ccw
  arc A979 (31.1498, 25.2094) -> (31.1498, 25.2856) centre (31.1498, 25.2475) ccw
  line L489 (22.4717, 25.2476) -> (21.1744, 25.2476)
  arc A980 (21.1744, 25.2857) -> (21.1744, 25.2095) centre (21.1744, 25.2476) ccw
  arc A981 (22.4717, 25.2095) -> (22.4717, 25.2857) centre (22.4717, 25.2476) ccw
  line L490 (31.1778, 25.3999) -> (29.8854, 25.4)
  arc A982 (29.8854, 25.4381) -> (29.8854, 25.3619) centre (29.8854, 25.4) ccw
  arc A983 (31.1778, 25.3618) -> (31.1778, 25.438) centre (31.1778, 25.3999) ccw
  line L491 (22.4386, 25.4) -> (21.1465, 25.4)
  arc A984 (21.1465, 25.4381) -> (21.1465, 25.3619) centre (21.1465, 25.4) ccw
  arc A985 (22.4386, 25.3619) -> (22.4386, 25.4381) centre (22.4386, 25.4) ccw
  line L492 (31.2051, 25.5524) -> (29.9186, 25.5524)
  arc A986 (29.9186, 25.5905) -> (29.9186, 25.5143) centre (29.9186, 25.5524) ccw
  arc A987 (31.2051, 25.5143) -> (31.2051, 25.5905) centre (31.2051, 25.5524) ccw
  line L493 (22.4054, 25.5524) -> (21.1189, 25.5524)
  arc A988 (21.1189, 25.5905) -> (21.1189, 25.5143) centre (21.1189, 25.5524) ccw
  arc A989 (22.4054, 25.5143) -> (22.4054, 25.5905) centre (22.4054, 25.5524) ccw
  line L494 (31.2139, 25.7047) -> (29.9389, 25.6983)
  arc A990 (29.9389, 25.7364) -> (29.9389, 25.6602) centre (29.9389, 25.6983) ccw
  arc A991 (31.2139, 25.6666) -> (31.2139, 25.7428) centre (31.2139, 25.7047) ccw
  line L495 (22.3847, 25.7048) -> (21.1097, 25.7048)
  arc A992 (21.1097, 25.7429) -> (21.1097, 25.6667) centre (21.1097, 25.7048) ccw
  arc A993 (22.3847, 25.6667) -> (22.3847, 25.7429) centre (22.3847, 25.7048) ccw
  line L496 (31.2224, 25.8572) -> (29.9502, 25.8572)
  arc A994 (29.9502, 25.8953) -> (29.9502, 25.8191) centre (29.9502, 25.8572) ccw
  arc A995 (31.2224, 25.8191) -> (31.2224, 25.8953) centre (31.2224, 25.8572) ccw
  line L497 (22.3738, 25.8572) -> (21.1004, 25.8572)
  arc A996 (21.1004, 25.8953) -> (21.1004, 25.8191) centre (21.1004, 25.8572) ccw
  arc A997 (22.3738, 25.8191) -> (22.3738, 25.8953) centre (22.3738, 25.8572) ccw
  line L498 (31.2308, 26.0096) -> (29.9611, 26.0096)
  arc A998 (29.9611, 26.0477) -> (29.9611, 25.9715) centre (29.9611, 26.0096) ccw
  arc A999 (31.2308, 25.9715) -> (31.2308, 26.0477) centre (31.2308, 26.0096) ccw
  line L499 (22.3629, 26.0096) -> (21.0912, 26.0096)
  arc A1000 (21.0912, 26.0477) -> (21.0912, 25.9715) centre (21.0912, 26.0096) ccw
  arc A1001 (22.3629, 25.9715) -> (22.3629, 26.0477) centre (22.3629, 26.0096) ccw
  line L500 (31.2392, 26.1619) -> (29.972, 26.162)
  arc A1002 (29.972, 26.2001) -> (29.972, 26.1239) centre (29.972, 26.162) ccw
  arc A1003 (31.2392, 26.1238) -> (31.2392, 26.2) centre (31.2392, 26.1619) ccw
  line L501 (22.352, 26.162) -> (21.082, 26.162)
  arc A1004 (21.082, 26.2001) -> (21.082, 26.1239) centre (21.082, 26.162) ccw
  arc A1005 (22.352, 26.1239) -> (22.352, 26.2001) centre (22.352, 26.162) ccw
  line L502 (31.2327, 26.3143) -> (29.9657, 26.3144)
  arc A1006 (29.9657, 26.3525) -> (29.9657, 26.2763) centre (29.9657, 26.3144) ccw
  arc A1007 (31.2327, 26.2762) -> (31.2327, 26.3524) centre (31.2327, 26.3143) ccw
  line L503 (22.352, 26.3144) -> (21.0956, 26.3144)
  arc A1008 (21.0956, 26.3525) -> (21.0956, 26.2763) centre (21.0956, 26.3144) ccw
  arc A1009 (22.352, 26.2763) -> (22.352, 26.3525) centre (22.352, 26.3144) ccw
  line L504 (31.2261, 26.4667) -> (29.9593, 26.4668)
  arc A1010 (29.9593, 26.5049) -> (29.9593, 26.4287) centre (29.9593, 26.4668) ccw
  arc A1011 (31.2261, 26.4286) -> (31.2261, 26.5048) centre (31.2261, 26.4667) ccw
  line L505 (22.3574, 26.4668) -> (21.1092, 26.4668)
  arc A1012 (21.1092, 26.5049) -> (21.1092, 26.4287) centre (21.1092, 26.4668) ccw
  arc A1013 (22.3574, 26.4287) -> (22.3574, 26.5049) centre (22.3574, 26.4668) ccw
  line L506 (31.2195, 26.6192) -> (29.953, 26.6192)
  arc A1014 (29.953, 26.6573) -> (29.953, 26.5811) centre (29.953, 26.6192) ccw
  arc A1015 (31.2195, 26.5811) -> (31.2195, 26.6573) centre (31.2195, 26.6192) ccw
  line L507 (22.3736, 26.6192) -> (21.1228, 26.6192)
  arc A1016 (21.1228, 26.6573) -> (21.1228, 26.5811) centre (21.1228, 26.6192) ccw
  arc A1017 (22.3736, 26.5811) -> (22.3736, 26.6573) centre (22.3736, 26.6192) ccw
  line L508 (31.2129, 26.7716) -> (29.9303, 26.7716)
  arc A1018 (29.9303, 26.8097) -> (29.9303, 26.7335) centre (29.9303, 26.7716) ccw
  arc A1019 (31.2129, 26.7335) -> (31.2129, 26.8097) centre (31.2129, 26.7716) ccw
  line L509 (22.3898, 26.7716) -> (21.1364, 26.7716)
  arc A1020 (21.1364, 26.8097) -> (21.1364, 26.7335) centre (21.1364, 26.7716) ccw
  arc A1021 (22.3898, 26.7335) -> (22.3898, 26.8097) centre (22.3898, 26.7716) ccw
  line L510 (31.1912, 26.924) -> (29.9038, 26.924)
  arc A1022 (29.9038, 26.9621) -> (29.9038, 26.8859) centre (29.9038, 26.924) ccw
  arc A1023 (31.1912, 26.8859) -> (31.1912, 26.9621) centre (31.1912, 26.924) ccw
  line L511 (22.406, 26.924) -> (21.1635, 26.924)
  arc A1024 (21.1635, 26.9621) -> (21.1635, 26.8859) centre (21.1635, 26.924) ccw
  arc A1025 (22.406, 26.8859) -> (22.406, 26.9621) centre (22.406, 26.924) ccw
  line L512 (31.1637, 27.0764) -> (29.8772, 27.0764)
  arc A1026 (29.8772, 27.1145) -> (29.8772, 27.0383) centre (29.8772, 27.0764) ccw
  arc A1027 (31.1637, 27.0383) -> (31.1637, 27.1145) centre (31.1637, 27.0764) ccw
  line L513 (22.4425, 27.0764) -> (21.1969, 27.0764)
  arc A1028 (21.1969, 27.1145) -> (21.1969, 27.0383) centre (21.1969, 27.0764) ccw
  arc A1029 (22.4425, 27.0383) -> (22.4425, 27.1145) centre (22.4425, 27.0764) ccw
  line L514 (31.1361, 27.2288) -> (29.8367, 27.2288)
  arc A1030 (29.8367, 27.2669) -> (29.8367, 27.1907) centre (29.8367, 27.2288) ccw
  arc A1031 (31.1361, 27.1907) -> (31.1361, 27.2669) centre (31.1361, 27.2288) ccw
  line L515 (22.4812, 27.2288) -> (21.2303, 27.2288)
  arc A1032 (21.2303, 27.2669) -> (21.2303, 27.1907) centre (21.2303, 27.2288) ccw
  arc A1033 (22.4812, 27.1907) -> (22.4812, 27.2669) centre (22.4812, 27.2288) ccw
  line L516 (31.1086, 27.3812) -> (29.789, 27.3812)
  arc A1034 (29.789, 27.4193) -> (29.789, 27.3431) centre (29.789, 27.3812) ccw
  arc A1035 (31.1086, 27.3431) -> (31.1086, 27.4193) centre (31.1086, 27.3812) ccw
  line L517 (22.5199, 27.3812) -> (21.2637, 27.3812)
  arc A1036 (21.2637, 27.4193) -> (21.2637, 27.3431) centre (21.2637, 27.3812) ccw
  arc A1037 (22.5199, 27.3431) -> (22.5199, 27.4193) centre (22.5199, 27.3812) ccw
  line L518 (31.0704, 27.5336) -> (29.7413, 27.5336)
  arc A1038 (29.7413, 27.5717) -> (29.7413, 27.4955) centre (29.7413, 27.5336) ccw
  arc A1039 (31.0704, 27.4955) -> (31.0704, 27.5717) centre (31.0704, 27.5336) ccw
  line L519 (22.5721, 27.5336) -> (21.3066, 27.5336)
  arc A1040 (21.3066, 27.5717) -> (21.3066, 27.4955) centre (21.3066, 27.5336) ccw
  arc A1041 (22.5721, 27.4955) -> (22.5721, 27.5717) centre (22.5721, 27.5336) ccw
  line L520 (31.0217, 27.686) -> (29.6795, 27.686)
  arc A1042 (29.6795, 27.7241) -> (29.6795, 27.6479) centre (29.6795, 27.686) ccw
  arc A1043 (31.0217, 27.6479) -> (31.0217, 27.7241) centre (31.0217, 27.686) ccw
  line L521 (22.635, 27.686) -> (21.3609, 27.686)
  arc A1044 (21.3609, 27.7241) -> (21.3609, 27.6479) centre (21.3609, 27.686) ccw
  arc A1045 (22.635, 27.6479) -> (22.635, 27.7241) centre (22.635, 27.686) ccw
  line L522 (30.9729, 27.8384) -> (29.6089, 27.8384)
  arc A1046 (29.6089, 27.8765) -> (29.6089, 27.8003) centre (29.6089, 27.8384) ccw
  arc A1047 (30.9729, 27.8003) -> (30.9729, 27.8765) centre (30.9729, 27.8384) ccw
  line L523 (22.6979, 27.8384) -> (21.4152, 27.8384)
  arc A1048 (21.4152, 27.8765) -> (21.4152, 27.8003) centre (21.4152, 27.8384) ccw
  arc A1049 (22.6979, 27.8003) -> (22.6979, 27.8765) centre (22.6979, 27.8384) ccw
  line L524 (30.9242, 27.9908) -> (29.5382, 27.9908)
  arc A1050 (29.5382, 28.0289) -> (29.5382, 27.9527) centre (29.5382, 27.9908) ccw
  arc A1051 (30.9242, 27.9527) -> (30.9242, 28.0289) centre (30.9242, 27.9908) ccw
  line L525 (22.7709, 27.9908) -> (21.4694, 27.9908)
  arc A1052 (21.4694, 28.0289) -> (21.4694, 27.9527) centre (21.4694, 27.9908) ccw
  arc A1053 (22.7709, 27.9527) -> (22.7709, 28.0289) centre (22.7709, 27.9908) ccw
  line L526 (30.8658, 28.1432) -> (29.449, 28.1432)
  arc A1054 (29.449, 28.1813) -> (29.449, 28.1051) centre (29.449, 28.1432) ccw
  arc A1055 (30.8658, 28.1051) -> (30.8658, 28.1813) centre (30.8658, 28.1432) ccw
  line L527 (22.8611, 28.1432) -> (21.5324, 28.1432)
  arc A1056 (21.5324, 28.1813) -> (21.5324, 28.1051) centre (21.5324, 28.1432) ccw
  arc A1057 (22.8611, 28.1051) -> (22.8611, 28.1813) centre (22.8611, 28.1432) ccw
  line L528 (30.7939, 28.2956) -> (29.3523, 28.2956)
  arc A1058 (29.3523, 28.3337) -> (29.3523, 28.2575) centre (29.3523, 28.2956) ccw
  arc A1059 (30.7939, 28.2575) -> (30.7939, 28.3337) centre (30.7939, 28.2956) ccw
  line L529 (22.9512, 28.2956) -> (21.6096, 28.2956)
  arc A1060 (21.6096, 28.3337) -> (21.6096, 28.2575) centre (21.6096, 28.2956) ccw
  arc A1061 (22.9512, 28.2575) -> (22.9512, 28.3337) centre (22.9512, 28.2956) ccw
  line L530 (30.7221, 28.448) -> (29.2552, 28.448)
  arc A1062 (29.2552, 28.4861) -> (29.2552, 28.4099) centre (29.2552, 28.448) ccw
  arc A1063 (30.7221, 28.4099) -> (30.7221, 28.4861) centre (30.7221, 28.448) ccw
  line L531 (23.0543, 28.448) -> (21.6867, 28.448)
  arc A1064 (21.6867, 28.4861) -> (21.6867, 28.4099) centre (21.6867, 28.448) ccw
  arc A1065 (23.0543, 28.4099) -> (23.0543, 28.4861) centre (23.0543, 28.448) ccw
  line L532 (30.6503, 28.6004) -> (29.1278, 28.6004)
  arc A1066 (29.1278, 28.6385) -> (29.1278, 28.5623) centre (29.1278, 28.6004) ccw
  arc A1067 (30.6503, 28.5623) -> (30.6503, 28.6385) centre (30.6503, 28.6004) ccw
  line L533 (23.1768, 28.6004) -> (21.7639, 28.6004)
  arc A1068 (21.7639, 28.6385) -> (21.7639, 28.5623) centre (21.7639, 28.6004) ccw
  arc A1069 (23.1768, 28.5623) -> (23.1768, 28.6385) centre (23.1768, 28.6004) ccw
  line L534 (30.5642, 28.7528) -> (29.0005, 28.7528)
  arc A1070 (29.0005, 28.7909) -> (29.0005, 28.7147) centre (29.0005, 28.7528) ccw
  arc A1071 (30.5642, 28.7147) -> (30.5642, 28.7909) centre (30.5642, 28.7528) ccw
  line L535 (23.2993, 28.7528) -> (21.8545, 28.7528)
  arc A1072 (21.8545, 28.7909) -> (21.8545, 28.7147) centre (21.8545, 28.7528) ccw
  arc A1073 (23.2993, 28.7147) -> (23.2993, 28.7909) centre (23.2993, 28.7528) ccw
  line L536 (30.4663, 28.9052) -> (28.8516, 28.9052)
  arc A1074 (28.8516, 28.9433) -> (28.8516, 28.8671) centre (28.8516, 28.9052) ccw
  arc A1075 (30.4663, 28.8671) -> (30.4663, 28.9433) centre (30.4663, 28.9052) ccw
  line L537 (23.4509, 28.9052) -> (21.9577, 28.9052)
  arc A1076 (21.9577, 28.9433) -> (21.9577, 28.8671) centre (21.9577, 28.9052) ccw
  arc A1077 (23.4509, 28.8671) -> (23.4509, 28.9433) centre (23.4509, 28.9052) ccw
  line L538 (30.3683, 29.0576) -> (28.6859, 29.0576)
  arc A1078 (28.6859, 29.0957) -> (28.6859, 29.0195) centre (28.6859, 29.0576) ccw
  arc A1079 (30.3683, 29.0195) -> (30.3683, 29.0957) centre (30.3683, 29.0576) ccw
  line L539 (23.6141, 29.0576) -> (22.061, 29.0576)
  arc A1080 (22.061, 29.0957) -> (22.061, 29.0195) centre (22.061, 29.0576) ccw
  arc A1081 (23.6141, 29.0195) -> (23.6141, 29.0957) centre (23.6141, 29.0576) ccw
  line L540 (30.2703, 29.21) -> (28.4999, 29.21)
  arc A1082 (28.4999, 29.2481) -> (28.4999, 29.1719) centre (28.4999, 29.21) ccw
  arc A1083 (30.2703, 29.1719) -> (30.2703, 29.2481) centre (30.2703, 29.21) ccw
  line L541 (23.7973, 29.21) -> (22.1643, 29.21)
  arc A1084 (22.1643, 29.2481) -> (22.1643, 29.1719) centre (22.1643, 29.21) ccw
  arc A1085 (23.7973, 29.1719) -> (23.7973, 29.2481) centre (23.7973, 29.21) ccw
  line L542 (30.1432, 29.3624) -> (28.2832, 29.3624)
  arc A1086 (28.2832, 29.4005) -> (28.2832, 29.3243) centre (28.2832, 29.3624) ccw
  arc A1087 (30.1432, 29.3243) -> (30.1432, 29.4005) centre (30.1432, 29.3624) ccw
  line L543 (24.0162, 29.3624) -> (22.2963, 29.3624)
  arc A1088 (22.2963, 29.4005) -> (22.2963, 29.3243) centre (22.2963, 29.3624) ccw
  arc A1089 (24.0162, 29.3243) -> (24.0162, 29.4005) centre (24.0162, 29.3624) ccw
  line L544 (30.0143, 29.5148) -> (28.0245, 29.5148)
  arc A1090 (28.0245, 29.5529) -> (28.0245, 29.4767) centre (28.0245, 29.5148) ccw
  arc A1091 (30.0143, 29.4767) -> (30.0143, 29.5529) centre (30.0143, 29.5148) ccw
  line L545 (24.2678, 29.5148) -> (22.4305, 29.5148)
  arc A1092 (22.4305, 29.5529) -> (22.4305, 29.4767) centre (22.4305, 29.5148) ccw
  arc A1093 (24.2678, 29.4767) -> (24.2678, 29.5529) centre (24.2678, 29.5148) ccw
  line L546 (29.8854, 29.6672) -> (27.7423, 29.6216)
  arc A1094 (27.7423, 29.6597) -> (27.7423, 29.5835) centre (27.7423, 29.6216) ccw
  arc A1095 (29.8854, 29.6291) -> (29.8854, 29.7053) centre (29.8854, 29.6672) ccw
  line L547 (24.5713, 29.6672) -> (22.5647, 29.6672)
  arc A1096 (22.5647, 29.7053) -> (22.5647, 29.6291) centre (22.5647, 29.6672) ccw
  arc A1097 (24.5713, 29.6291) -> (24.5713, 29.7053) centre (24.5713, 29.6672) ccw
  line L548 (29.7304, 29.8196) -> (27.563, 29.2165)
  arc A1098 (27.563, 29.2546) -> (27.563, 29.1784) centre (27.563, 29.2165) ccw
  arc A1099 (29.7304, 29.7815) -> (29.7304, 29.8577) centre (29.7304, 29.8196) ccw
  line L549 (25.0026, 29.8196) -> (22.7253, 29.8196)
  arc A1100 (22.7253, 29.8577) -> (22.7253, 29.7815) centre (22.7253, 29.8196) ccw
  arc A1101 (25.0026, 29.7815) -> (25.0026, 29.8577) centre (25.0026, 29.8196) ccw
  line L550 (29.5628, 29.972) -> (27.3473, 28.2614)
  arc A1102 (27.3093, 28.2639) -> (27.3473, 28.2233) centre (27.3473, 28.2614) ccw
  arc A1103 (29.5628, 29.9339) -> (29.5628, 30.0101) centre (29.5628, 29.972) ccw
  line L551 (26.162, 29.972) -> (22.8983, 29.972)
  arc A1104 (22.8983, 30.0101) -> (22.8983, 29.9339) centre (22.8983, 29.972) ccw
  arc A1105 (26.162, 29.9339) -> (26.162, 30.0101) centre (26.162, 29.972) ccw
  line L552 (29.3951, 30.1244) -> (-0.9498, 30.1244)
  arc A1106 (-0.9878, 30.1269) -> (-0.9118, 30.1219) centre (-0.9498, 30.1244) ccw
  arc A1107 (29.3951, 30.0863) -> (29.3951, 30.1625) centre (29.3951, 30.1244) ccw
  line L553 (26.162, 30.1244) -> (23.0714, 30.1244)
  arc A1108 (23.0714, 30.1625) -> (23.0714, 30.0863) centre (23.0714, 30.1244) ccw
  arc A1109 (26.162, 30.0863) -> (26.162, 30.1625) centre (26.162, 30.1244) ccw
  line L554 (27.2302, 31.122) -> (27.0432, 28.2814)
  arc A1110 (27.0052, 28.2839) -> (27.0812, 28.2789) centre (27.0432, 28.2814) ccw
  arc A1111 (27.2302, 31.0839) -> (27.2302, 31.1601) centre (27.2302, 31.122) ccw
  line L555 (26.162, 30.2768) -> (23.2868, 30.2768)
  arc A1112 (23.2868, 30.3149) -> (23.2868, 30.2387) centre (23.2868, 30.2768) ccw
  arc A1113 (26.162, 30.2387) -> (26.162, 30.3149) centre (26.162, 30.2768) ccw
  line L556 (27.1241, 30.7326) -> (21.4917, 28.6469)
  arc A1114 (21.4537, 28.6494) -> (21.5298, 28.6444) centre (21.4917, 28.6469) ccw
  arc A1115 (27.1241, 30.6945) -> (27.1241, 30.7707) centre (27.1241, 30.7326) ccw
  line L557 (26.162, 30.4292) -> (23.5117, 30.4292)
  arc A1116 (23.5117, 30.4673) -> (23.5117, 30.3911) centre (23.5117, 30.4292) ccw
  arc A1117 (26.162, 30.3911) -> (26.162, 30.4673) centre (26.162, 30.4292) ccw
  line L558 (26.8955, 30.6777) -> (26.7391, 28.3014)
  arc A1118 (26.701, 28.3039) -> (26.7771, 28.2989) centre (26.7391, 28.3014) ccw
  arc A1119 (26.8955, 30.6396) -> (26.8955, 30.7158) centre (26.8955, 30.6777) ccw
  line L559 (26.162, 30.5816) -> (23.7661, 30.5816)
  arc A1120 (23.7661, 30.6197) -> (23.7661, 30.5435) centre (23.7661, 30.5816) ccw
  arc A1121 (26.162, 30.5435) -> (26.162, 30.6197) centre (26.162, 30.5816) ccw
  line L560 (26.724, 30.3927) -> (26.587, 28.3115)
  arc A1122 (26.549, 28.314) -> (26.625, 28.309) centre (26.587, 28.3115) ccw
  arc A1123 (26.724, 30.3546) -> (26.724, 30.4308) centre (26.724, 30.3927) ccw
  line L561 (26.162, 30.734) -> (24.067, 30.734)
  arc A1124 (24.067, 30.7721) -> (24.067, 30.6959) centre (24.067, 30.734) ccw
  arc A1125 (26.162, 30.6959) -> (26.162, 30.7721) centre (26.162, 30.734) ccw
  line L562 (26.5493, 30.0586) -> (26.4349, 28.3215)
  arc A1126 (26.3969, 28.324) -> (26.4729, 28.319) centre (26.4349, 28.3215) ccw
  arc A1127 (26.5493, 30.0205) -> (26.5493, 30.0967) centre (26.5493, 30.0586) ccw
  line L563 (26.162, 30.8864) -> (24.4226, 30.8864)